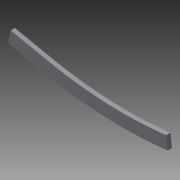
# Autodesk Inventor part: nd-11
Saved by Autodesk Inventor 2015 (Build 190159000, 159)
## iProperties
Created: 2014-07-02
Part Number: nd-11
Material: Generic
Document SubType Name: Modeling
Designer: peter
Density: 1 g/cm^3
Appearance: Default
Author: peter
Autodesk Inventor part; units mm, degrees
ref_plane "YZ Plane" through (0, 0, 0) normal (1, 0, 0) x (0, 1, 0)
ref_plane "XZ Plane" through (0, 0, 0) normal (0, 1, 0) x (-1, 0, 0)
ref_plane "XY Plane" through (0, 0, 0) normal (0, 0, 1) x (1, 0, 0)
sketch "Sketch1" plane through (0, 0, 0) normal (0, 0, 1) x (1, 0, 0)
  line L0 (17.895, 126.526) -> (6.2291, 70.5793)
  line L1 (6.2291, 70.5793) -> (180.4099, 34.2593)
  line L2 (180.4099, 34.2593) -> (180.4999, 34.2409)
  arc A0 (180.4999, 34.2409) -> (729.8636, 11.0979) centre (526.9522, 1726.3374) ccw
  line L3 (729.8636, 11.0979) -> (723.1497, 67.8521)
  arc A1 (191.9747, 90.2271) -> (723.1497, 67.8521) centre (526.9522, 1726.3374) ccw
  line L4 (191.9747, 90.2271) -> (17.895, 126.526)
  point P0 (0, 0)
  constraints: 10 end point, 4 point on circle, 2 centre point
extrude "Extrusion1" add sketch "Sketch1" along normal blind 19.05
body "Solid1"
